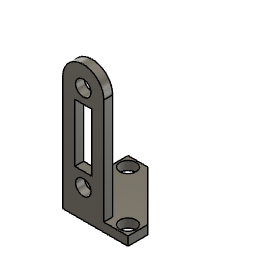
limit_mount_v5 (Autodesk Fusion 360 design; units mm, degrees)
Autodesk Fusion 360 part; units mm, degrees
note: some values were not read from the file. Chosen so that the rebuilt part matches the saved one: which face or edge a step refers to. Set by a fixed rule: which sketch regions a step uses.
sketch "Sketch1" plane through (0, 0, 0) normal (0, 1, 0) x (1, 0, 0)
  circle A0 centre (0, 0) radius 1.85
  circle A1 centre (11.3137, -11.3137) radius 1.85
  line L0 (11.3137, -11.3137) -> (14.4887, -11.3137) construction
  line L1 (-2.2451, -2.2451) -> (-2.2451, 2.2451)
  line L2 (9.0686, -13.5588) -> (13.5588, -13.5588)
  line L3 (2.2451, 2.2451) -> (-2.2451, 2.2451)
  line L4 (13.5588, -9.0686) -> (13.5588, -13.5588)
  line L5 (13.5588, -9.0686) -> (2.2451, 2.2451)
  line L6 (9.0686, -13.5588) -> (-2.2451, -13.5588)
  line L7 (0, -13.5588) -> (7, -13.5588)
  line L8 (-2.2451, -13.5588) -> (-2.2451, -11.5588)
  line L9 (-2.2451, -11.5588) -> (7.0686, -11.5588)
  line L10 (-2.2451, -13.5588) -> (-2.2451, -11.5588)
  line L11 (-2.2451, -2.2451) -> (7.0686, -11.5588)
  line L12 (7.0686, -11.5588) -> (9.0686, -13.5588)
  line L13 (-2.2451, -11.5588) -> (-2.2451, -2.2451)
  dimension "d1" = 16
  dimension "d2" = 3.7
  dimension "d3" = 3.7
  dimension "d5" = 3.175
  dimension "d8" = 3.175
  dimension "d15" = 3.175
  dimension "d18" = 2
  constraint coincident A0.centre origin
  constraint horizontal L0
  constraint coincident A1.centre L0.start
  constraint vertical L1
  constraint perpendicular L1 L6
  constraint coincident L6 L7.start
  constraint coincident L6 L7.end
  constraint perpendicular L6 L8
  constraint perpendicular L9 L10
  constraint perpendicular L9 L13
  measures "d1" distance of A0.centre A1.centre
  measures "d2" diameter of A0
  measures "d3" diameter of A1
  measures "d5" distance of A0.centre L1.start
  measures "d8" distance of A1.centre L2.start
  measures "d15" distance of A0.centre L1.end
  measures "d18" distance of L6.end L8.end
extrude "Extrude5" add sketch "Sketch1" along normal blind 2 contours L9 L11 L13 makes body 1
extrude "Extrude2" add sketch "Sketch1" along normal blind 26 separate body contours L6 L7 L8 L9 L10 L12 makes body 2
extrude "Extrude1" add sketch "Sketch1" along normal blind 2 separate body contours L1 L2 L3 L4 L5 L11 L12 makes body 3
sketch "Sketch2" plane through (0, 0, 13.5588) normal (0, 0, 1) x (1, 0, 0)
  line L0 (-2.2451, 0) -> (9.0686, 0)
  line L1 (9.0686, 0) -> (9.0686, 26)
  line L2 (9.0686, 26) -> (-2.2451, 26)
  line L3 (-2.2451, 26) -> (-2.2451, 0)
  line L4 (3.4118, 0) -> (3.4118, 4)
  line L5 (3.4118, 6.5) -> (3.4118, 26)
  circle A0 centre (3.4118, 26) radius 1.75
  arc A1 (9.0686, 26) -> (-2.2451, 26) centre (3.4118, 26) ccw
  circle A2 centre (3.4118, 6.5) radius 1.75
  dimension "d24" = 4
  dimension "d26" = 19.5
  dimension "d27" = 3.5
  dimension "d39" = 3.5
  constraint midpoint L0 L4.start
  constraint perpendicular L0 L4
  constraint coincident L5.end A0.centre
  constraint coincident L5.start A2.centre
  measures "d24" distance of L4.start L4.end
  measures "d26" distance of L5.start L5.end
  measures "d27" diameter of A0
  measures "d39" diameter of A2
extrude "Extrude9" cut sketch "Sketch2" against normal blind 2 contours A2 bodies 2
extrude "Extrude4" cut sketch "Sketch2" against normal blind 2 contours L0 L1 L2 L3 A0 | L2 A0 | L2 L5 A0 | L2 L5 A0 bodies 2
extrude "Extrude3" add sketch "Sketch2" against normal blind 2 contours L2 A0 A1 bodies 2
extrude "Extrude6" cut 1 faces at (7.7664, 26, 12.8921) along direction (0, 1, 0) blind 9 on bodies 2 bodies 2
sketch "Sketch3" plane through (0, 0, 13.5588) normal (0, 0, 1) x (1, 0, 0)
  line L0 (3.4118, 26) -> (3.4118, 5.7496)
  line L1 (5.5617, 8.3524) -> (1.2619, 8.3524)
  line L2 (1.2619, 8.3524) -> (1.2619, 23.3972)
  line L3 (1.2619, 23.3972) -> (5.5617, 23.3972)
  line L4 (5.5617, 23.3972) -> (5.5617, 8.3524)
  line L5 (5.5617, 8.3524) -> (1.2619, 23.3972) construction
  line L6 (1.2619, 8.3524) -> (5.5617, 23.3972) construction
  point P0 (3.4118, 26)
  point P1 (3.4118, 5.7496)
  point P2 (3.4118, 15.8748)
  constraint coincident P0 L0.start
  constraint coincident P1 L0.end
  constraint horizontal L1
  constraint perpendicular L1 L2
  constraint parallel L1 L3
  constraint parallel L2 L4
  constraint coincident L5 P2
  constraint coincident L6 P2
  constraint midpoint L0 P2
extrude "Extrude7" cut sketch "Sketch3" against normal blind 6 bodies 2
extrude "Extrude8" add sketch "Sketch2" against normal blind 2 contours L0 L1 L2 L3 A0 | L2 A0 A1 bodies 3 1 2
move_face "OffsetFaces1" offset -1 3 faces at (-2.2451, 9.3333, 12.8921) (9.0686, 18, 12.2254) (9.0405, 26.5632, 12.2254) on bodies 3
sketch "Sketch4" plane through (0, 0, 13.5588) normal (0, 0, 1) x (1, 0, 0)
  line L0 (5.3426, 9.6599) -> (1.4809, 9.6599)
  line L1 (1.4809, 9.6599) -> (1.4809, 22.8401)
  line L2 (1.4809, 22.8401) -> (5.3426, 22.8401)
  line L3 (5.3426, 22.8401) -> (5.3426, 9.6599)
  line L4 (5.3426, 9.6599) -> (1.4809, 22.8401) construction
  line L5 (1.4809, 9.6599) -> (5.3426, 22.8401) construction
  line L6 (3.4118, 6.5) -> (3.4118, 26)
  point P0 (3.4118, 16.25)
  constraint horizontal L0
  constraint perpendicular L0 L1
  constraint parallel L0 L2
  constraint parallel L1 L3
  constraint coincident L4 P0
  constraint coincident L5 P0
  constraint midpoint P0 L6
extrude "Extrude10" cut sketch "Sketch4" against normal blind 2 bodies 3
extrude "Extrude11" add sketch "Sketch1" along normal blind 2 contours L1 L2 L3 L4 L5 L11 L12 | L9 L11 L13 bodies 3
chamfer "Chamfer1" distance 1 angle 45 1 edges at (-2.2451, 1, 11.5588) on bodies 3
